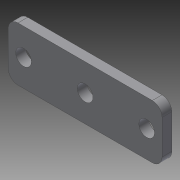
# Autodesk Inventor part: Vertical_Lead_Screw_E-stop_Plate
Saved by Autodesk Inventor 2015 (Build 190159000, 159)
## iProperties
Created: 2015-01-06
Part Number: Vertical_Lead_Screw_E-stop_Plate
Material: Generic
Document SubType Name: Modeling
Designer: Drew
Density: 1 g/cm^3
Appearance: Default
Author: Drew
Autodesk Inventor part; units mm, degrees
ref_plane "YZ Plane" through (0, 0, 0) normal (1, 0, 0) x (0, 1, 0)
ref_plane "XZ Plane" through (0, 0, 0) normal (0, 1, 0) x (-1, 0, 0)
ref_plane "XY Plane" through (0, 0, 0) normal (0, 0, 1) x (1, 0, 0)
sketch "Sketch1" plane through (0, 0, 0) normal (0, 0, 1) x (1, 0, 0)
  line L0 (43.65, -17.5) -> (-43.65, -17.5)
  line L1 (-50, -11.15) -> (-50, 11.15)
  line L2 (-43.65, 17.5) -> (43.65, 17.5)
  line L3 (50, 11.15) -> (50, -11.15)
  line L4 (50, -17.5) -> (-50, 17.5) construction
  line L5 (-50, -17.5) -> (50, 17.5) construction
  line L6 (0, 51.2558) -> (0, -45.9758)
  circle A0 centre (-40, 0) radius 5.1
  line L7 (-83.6339, 0) -> (65.0593, 0)
  circle A1 centre (40, 0) radius 5.1
  circle A2 centre (0, 0) radius 5.1
  arc A3 (-43.65, 17.5) -> (-50, 11.15) centre (-43.65, 11.15) ccw
  arc A4 (-50, -11.15) -> (-43.65, -17.5) centre (-43.65, -11.15) ccw
  arc A5 (43.65, -17.5) -> (50, -11.15) centre (43.65, -11.15) ccw
  arc A6 (50, 11.15) -> (43.65, 17.5) centre (43.65, 11.15) ccw
  point P0 (0, 0)
  point P1 (0, 0)
  dimension "d0" = 100
  dimension "d1" = 35
  dimension "d2" = 80
  dimension "d3" = 10.2
  dimension "d6" = 10.2
  dimension "d7" = 6.35
  constraints: 16 end point, 11 point on line, 8 point on circle, 8 tangent, 7 centre point, 4 midpoint, 3 equal radius, 2 horizontal, 2 parallel, 1 coincident, 1 perpendicular, 1 symmetric about line, 1 vertical, 1 other
  measures "d0" distance of L4.end L5.end
  measures "d1" distance of L5.start L4.end
  measures "d2" diameter of A0.centre L6
  measures "d3" diameter of A0
  measures "d6" diameter of A2
  measures "d7" radius of A3
extrude "Extrusion1" add sketch "Sketch1" along normal blind 6.35 contours L0 L6 A2 L7 A1 L3 A5 | L0 A4 L1 L7 A0 A2 L6 | L7 A1 A2 L6 L2 A6 L3 | L7 A0 L1 A3 L2 L6 A2
equation "\"d6\" = d3"
body "Solid1"
